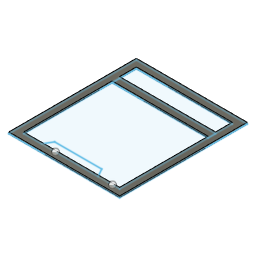
Switch Film v3 (Autodesk Fusion 360 design; units mm, degrees)
Autodesk Fusion 360 part; units mm, degrees
sketch "Sketch1" plane through (0, 0, 0) normal (0, 0, 1) x (1, 0, 0)
  line L0 (-12.0522, 11.3823) -> (-1.7522, 11.3823)
  line L1 (-1.7522, 11.3823) -> (-1.7522, -0.7177)
  line L2 (-1.7522, -0.7177) -> (-12.0522, -0.7177)
  line L3 (-12.0522, -0.7177) -> (-12.0522, 11.3823)
  line L4 (-0.9522, -1.5177) -> (-12.8522, -1.5177)
  line L5 (-12.8522, -1.5177) -> (-12.8522, 12.1823)
  line L6 (-12.8522, 12.1823) -> (-0.9522, 12.1823)
  line L7 (-0.9522, 12.1823) -> (-0.9522, -1.5177)
  line L8 (-12.0522, 9.5823) -> (-1.7522, 9.5823)
  line L9 (-1.7522, 9.5823) -> (-1.7522, 8.7823)
  line L10 (-1.7522, 8.7823) -> (-12.0522, 8.7823)
  line L11 (-12.0522, 8.7823) -> (-12.0522, 9.5823)
  line L12 (-10.1522, -0.7177) -> (-9.6325, 0.1823)
  line L13 (-10.1522, -0.7177) -> (-8.6478, -0.7177) construction
  line L14 (-4.059, -0.7177) -> (-4.5786, 0.1823)
  line L15 (-4.059, -0.7177) -> (-2.5223, -0.7177) construction
  line L16 (-9.6325, 0.1823) -> (-4.5786, 0.1823)
  dimension "d1" = 12.1
  dimension "d2" = 10.3
  dimension "d3" = -0.8
  dimension "d4" = 0.8
  dimension "d5" = 1.8
  dimension "d6" = 60
  dimension "d7" = 0.9
  dimension "d11" = 0.9
  dimension "d12" = 60
  dimension "d19" = 1.9
  dimension "d20" = 10.3
  constraint horizontal L0
  constraint vertical L1
  constraint horizontal L2
  constraint vertical L3
  constraint horizontal L8
  constraint vertical L9
  constraint horizontal L10
  constraint vertical L11
  constraint coincident L3 L8.start
  constraint horizontal L13
  constraint coincident L2 L12.start
  constraint horizontal L15
  constraint coincident L2 L14.start
  measures "d1" distance of L0.start L2.end
  measures "d2" distance of L0.start L0.end
  measures "d4" distance of L8.start L10.end
  measures "d5" distance of L0 L8
  measures "d6" angle of L12 L13
  measures "d7" distance of L12.end L13
  measures "d11" distance of L2 L14.end
  measures "d12" angle of L2 L14
  measures "d19" distance of L2.end L12.start
  measures "d20" distance of L3 L9
extrude "Extrude1" add sketch "Sketch1" along normal blind 0.16
extrude "Extrude2" add sketch "Sketch1" along normal blind 0.16 contours L1 L3 L8 L9 L10 L11
